Bottom Bearing_v1 (Autodesk Fusion 360 design; units mm, degrees)
Autodesk Fusion 360 part; units mm, degrees
sketch "Sketch1" plane through (0, 0, 0) normal (0, 0, 1) x (1, 0, 0)
  circle A0 centre (0, 0) radius 34.5
  circle A1 centre (0, 0) radius 23
  dimension "d1" = 69
  dimension "d2" = 46
  constraint coincident A0.centre A1.centre
  constraint concentric A0 A1
  measures "d1" diameter of A0
  measures "d2" diameter of A1
extrude "Extrude1" add sketch "Sketch1" along normal blind 11 makes body 1
sketch "Sketch4" plane through (0, 0, 11) normal (0, 0, 1) x (-1, 0, 0)
  circle A0 centre (0, 0) radius 23
  circle A1 centre (0, 0) radius 34.5
  circle A2 centre (0, 0) radius 32.5
  dimension "d27" = 65
  constraint coincident A0.centre A1.centre
  measures "d27" diameter of A2
extrude "Extrude5" cut sketch "Sketch4" against normal blind 9 contours A1 bodies 1
sketch "Sketch2" plane through (0, 0, 11) normal (0, 0, 1) x (-1, 0, 0)
  circle A0 centre (0, 0) radius 23
  circle A1 centre (0, 0) radius 28 construction
  circle A2 centre (0, -28) radius 2
  circle A3 centre (0, -28) radius 4.0625
  circle A4 centre (0, 0) radius 32.5
  dimension "d12" = 56
  dimension "d13" = 4
  dimension "d14" = 8.125
  constraint coincident A0.centre A1.centre
  constraint coincident A1 A2.centre
  constraint concentric A2 A3
  measures "d12" diameter of A1
  measures "d13" diameter of A2
  measures "d14" diameter of A3
extrude "Extrude2" cut sketch "Sketch2" against normal blind 22 contours A2 bodies 1
extrude "Extrude3" add sketch "Sketch2" along normal blind 7 contours A3 bodies 1
chamfer "Chamfer1" distance 6 angle 45 1 edges at (3.7876, 26.5309, 11) on bodies 1
sketch "Sketch3" plane through (0, 0, 0) normal (0, 0, -1) x (1, 0, 0)
  circle A0 centre (0, -28) radius 2
  circle A1 centre (0, 0) radius 23
  circle A2 centre (0, 0) radius 34.5
  line L0 (4.0067, -28.03) -> (2.0294, -24.5451)
  line L1 (2.0294, -24.5451) -> (-1.9773, -24.5151)
  line L2 (-1.9773, -24.5151) -> (-4.0067, -27.97)
  line L3 (-4.0067, -27.97) -> (-2.0294, -31.4549)
  line L4 (-2.0294, -31.4549) -> (1.9773, -31.4849)
  line L5 (1.9773, -31.4849) -> (4.0067, -28.03)
  point P0 (0, -28)
  dimension "d20" = 3.47
  constraint coincident P0 A0.centre
  measures "d20" distance of P0 L5
extrude "Extrude4" cut sketch "Sketch3" against normal blind 5 contours L0 L1 L2 L3 L4 L5 bodies 1
pattern_circular "C-Pattern1" count 5 over 360 about axis through (0, 0, 1.75) along (0, 0, 1) of "Extrude2", "Extrude3", "Chamfer1", "Extrude4"
copy_body "Body->Comp1" bodies 1 removing the originals makes body 2 in component "OutputShaft Bottom"
copy_body "CopyPasteBodies1" [suppressed]
extrude "Extrude1'" [suppressed] in component "OutputShaft Bottom"
extrude "Extrude2'" [suppressed] in component "OutputShaft Bottom"
move_face "OffsetFaces1" [suppressed] in component "OutputShaft Bottom"
sketch "Sketch5" plane through (0, 0, 11) normal (0, 0, 1) x (-1, 0, 0)
  arc A0 (-111.0097, 19.4871) -> (-95.4959, 30.7585) centre (-101.458, 22.6525) ccw
  arc A1 (-111.0097, 19.4871) -> (-117.4965, -0.4773) centre (-85, 0) ccw
  arc A2 (-111.5708, -18.7148) -> (-117.4965, -0.4773) centre (-111.6296, -8.6525) ccw
  arc A3 (-111.5708, -18.7148) -> (-94.588, -31.0535) centre (-85, 0) ccw
  arc A4 (-75.412, -31.0535) -> (-94.588, -31.0535) centre (-85, -28) ccw
  arc A5 (-75.412, -31.0535) -> (-58.4292, -18.7148) centre (-85, 0) ccw
  arc A6 (-52.5035, -0.4773) -> (-58.4292, -18.7148) centre (-58.3704, -8.6525) ccw
  arc A7 (-52.5035, -0.4773) -> (-58.9903, 19.4871) centre (-85, 0) ccw
  arc A8 (-74.5041, 30.7585) -> (-58.9903, 19.4871) centre (-68.542, 22.6525) ccw
  arc A9 (-74.5041, 30.7585) -> (-95.4959, 30.7585) centre (-85, 0) ccw
  circle A10 centre (-85, 0) radius 13
sketch "Sketch6" plane through (0, 0, 11) normal (0, 0, 1) x (-1, 0, 0)
  circle A0 centre (-85, 0) radius 16
  point P0 (-85, 0)
  dimension "d35" = 32
  constraint coincident P0 A0.centre
  measures "d35" diameter of A0
extrude "Extrude3'" [suppressed] in component "OutputShaft Bottom"
component "OutputShaft Bottom" placed x (1, 0, 0) y (0, 1, 0) z (0, 0, 1) at (85, 0, 0)
equation "d1 = OuterLipDia"
equation "d2 = InnerBearingDia"
equation "InnerBearingDia = 46 mm"
equation "OuterLipDia = 69 mm"
equation "OuterBearingDia = 65 mm"
equation "Height = 11 mm"
equation "d7 = Height"
equation "BoltDia = 4 mm"
equation "BoltWall = 8.125 mm"
equation "BoltHoleRad = 28 mm"
equation "d12 = BoltHoleRad * 2"
equation "d13 = BoltDia"
equation "d14 = BoltWall"
equation "d20 = BoltHeadDia"
equation "d21 = BoltHeadDepth"
equation "BoltHeadDia = 3.47 mm"
equation "BoltHeadDepth = -5 mm"
equation "d27 = OuterBearingDia"
equation "OuterBearingHeight = -9 mm"
